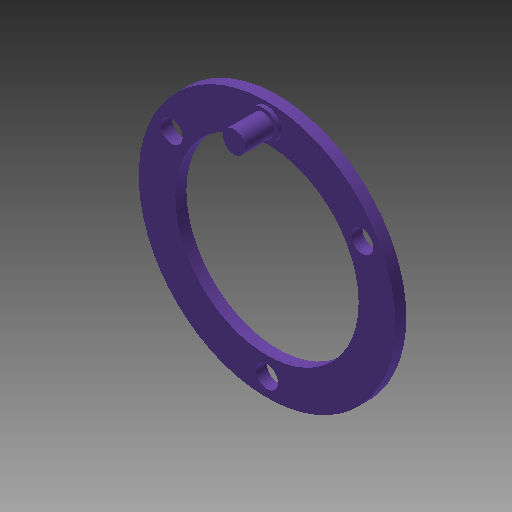
# Autodesk Inventor part: Ring1
Saved by Autodesk Inventor 2019 (Build 230136000, 136)
## iProperties
Created: 2017-01-18
Part Number: Ring1
Document SubType Name: Modeling
Designer: Administrator
Density: 1 g/cm^3
Mass: 5.67686 g
Surface Area: 50.7681 cm^2
Volume: 5.67686 cm^3
Material: Generic
Appearance: Violet
Author: Administrator
Autodesk Inventor part; units mm, degrees
ref_plane "YZ Plane" through (0, 0, 0) normal (1, 0, 0) x (0, 1, 0)
ref_plane "XZ Plane" through (0, 0, 0) normal (0, 1, 0) x (-1, 0, 0)
ref_plane "XY Plane" through (0, 0, 0) normal (0, 0, 1) x (1, 0, 0)
sketch "Sketch1" plane through (0, 0, 0) normal (0, 0, 1) x (1, 0, 0)
  circle A0 centre (0, 0) radius 30 construction
  line L0 (0, 0) -> (0, 7.5) construction
  line L1 (0, 7.5) -> (10, 7.5) construction
  line L2 (10, 7.5) -> (10, 0) construction
  line L3 (10, 0) -> (0, 0) construction
  line L4 (0, 0) -> (-10, 0) construction
  line L5 (-10, 0) -> (-10, 7.5) construction
  line L6 (-10, 7.5) -> (0, 7.5) construction
  line L7 (-10, 0) -> (-10, -7.5) construction
  line L8 (-10, -7.5) -> (10, -7.5) construction
  line L9 (10, -7.5) -> (10, 0) construction
  circle A1 centre (-15.5891, 25.6316) radius 10 construction
  circle A2 centre (0, 0) radius 35
  circle A3 centre (0, 0) radius 25
  line L10 (0, 0) -> (-31.8198, 31.8198) construction
  circle A4 centre (0, 0) radius 45 construction
  line L11 (0, 0) -> (0, 45) construction
  circle A5 centre (0, 0) radius 40 construction
  circle A6 centre (-40, 0) radius 5 construction
  circle A7 centre (-31.8198, 31.8198) radius 10 construction
  line L12 (-31.8198, 31.8198) -> (-31.8198, -24.2384) construction
  line L13 (-31.8198, -24.2384) -> (-31.8198, -31.8198) construction
  circle A8 centre (-31.8198, -31.8198) radius 10 construction
  line L14 (-15, -20) -> (-15, -31.6228) construction
  line L15 (15, -20) -> (15, -31.6228) construction
  line L16 (-31.8198, 31.8198) -> (24.2384, 31.8198) construction
  line L17 (24.2384, 31.8198) -> (31.8198, 31.8198) construction
  line L18 (31.8198, 31.8198) -> (31.8198, -31.8198) construction
  line L19 (31.8198, -31.8198) -> (-31.8198, -31.8198) construction
  circle A9 centre (31.8198, 31.8198) radius 10 construction
  circle A10 centre (31.8198, -31.8198) radius 10 construction
  circle A11 centre (0, 40) radius 5 construction
  line L20 (0, 0) -> (40, 0) construction
  line L21 (0, 0) -> (0, -40) construction
  circle A12 centre (40, 0) radius 5 construction
  circle A13 centre (0, -40) radius 5 construction
  line L22 (50, 50) -> (50, -50) construction
  line L23 (50, -50) -> (-50, -50) construction
  line L24 (-50, -50) -> (-50, 50) construction
  line L25 (-50, 50) -> (50, 50) construction
  circle A14 centre (0, 30) radius 3
  point P0 (0, 50)
  dimension "d9" = 80
  dimension "d0" = 60
  dimension "d1" = 20
  dimension "d2" = 15
  dimension "d3" = 20
  dimension "d4" = 5
  dimension "d5" = 5
  dimension "d6" = 90
  dimension "d7" = 45
  dimension "d10" = 10
  dimension "d12" = 20
  dimension "d13" = 15
  dimension "d14" = 100
  dimension "d15" = 6
  constraints: 52 end point, 12 centre point, 9 coincident, 9 parallel, 7 perpendicular, 7 point on circle, 5 collinear, 3 point on line, 2 symmetric about line, 1 midpoint, 1 vertical, 29 other
  measures "d0" diameter of A0
  measures "d1" distance of L7.end L8.end
  measures "d2" distance between parallel lines of L8 L6
  measures "d3" diameter of A1
  measures "d6" diameter of A4
  measures "d7" angle of L11 L10
  measures "d10" diameter of A6
  measures "d12" diameter of A7
  measures "d13" distance between parallel lines of L14 L11
  measures "d14" distance of L22.start L22.end
  measures "d15" diameter of A14
extrude "Extrusion1" add sketch "Sketch1" along normal blind 3
sketch "Sketch2" plane through (0, 0, 0) normal (0, 0, -1) x (-1, 0, 0)
  circle A0 centre (0, 30) radius 3 projected
extrude "Extrusion2" add sketch "Sketch2" against normal blind 12
sketch "Sketch3" plane through (0, 0, 3) normal (0, 0, 1) x (1, 0, 0)
  circle A0 centre (0, 30) radius 3 projected
  circle A1 centre (0, 30) radius 4
  dimension "d20" = 8
  constraints: 1 centre point
  measures "d20" diameter of A1
extrude "Extrusion3" add sketch "Sketch3" along normal blind 1
sketch "Sketch4" plane through (0, 0, 3) normal (0, 0, 1) x (1, 0, 0)
  circle A0 centre (0, 0) radius 25 projected
  circle A1 centre (0, 0) radius 35 projected
  line L0 (0, 0) -> (0, -25) construction
  line L1 (0, -25) -> (0, -35) construction
  circle A2 centre (0, -30) radius 3
  dimension "d23" = 6
  constraints: 4 end point, 2 vertical alignment, 1 centre point, 1 collinear, 1 midpoint, 1 vertical, 2 other
  measures "d23" diameter of A2
extrude "Extrusion4" cut sketch "Sketch4" against normal blind 10 contours A2
pattern_circular "Circular Pattern1" count 3 over 360 about axis through (0, 0, -10) along (0, 0, 1) of "Extrusion4"
body "Solid1"
